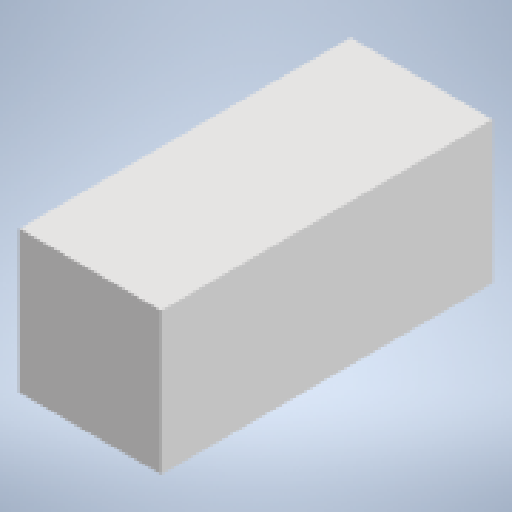
# Autodesk Inventor part: CalibrationPlate
Saved by Autodesk Inventor 2024 (Build 280153000, 153)
## iProperties
Created: 2023-12-31
Part Number: CalibrationPlate
Material: Generic
Document SubType Name: Modeling
Designer: jevan
Density: 1 g/cm^3
Appearance: Default
Author: jevan
Autodesk Inventor part; units mm, degrees
ref_plane "YZ Plane" through (0, 0, 0) normal (1, 0, 0) x (0, 1, 0)
ref_plane "XZ Plane" through (0, 0, 0) normal (0, 1, 0) x (-1, 0, 0)
ref_plane "XY Plane" through (0, 0, 0) normal (0, 0, 1) x (1, 0, 0)
sketch "Sketch1" plane through (0, 0, 0) normal (0, 1, 0) x (-1, 0, 0)
  line L0 (0, 0) -> (30, 0)
  line L1 (30, 0) -> (30, -70)
  line L2 (30, -70) -> (0, -70)
  line L3 (0, -70) -> (0, 0)
  dimension "d0" = 70
  dimension "d1" = 30
  constraints: 8 end point, 2 parallel, 1 horizontal, 1 perpendicular
  measures "d0" distance between parallel lines of L0 L2
  measures "d1" distance between parallel lines of L3 L1
extrude "Extrusion1" add sketch "Sketch1" along normal blind 30
sketch "Sketch2" plane through (0, 30, 0) normal (0, 1, 0) x (1, 0, 0)
  line L0 (-30, 70) -> (-30, 0) projected
  line L1 (0, 70) -> (-30, 70) projected
  line L2 (-30, 0) -> (0, 0)
  line L3 (0, 0) -> (0, 70)
  line L4 (0, 70) -> (-30, 70)
  line L5 (-30, 70) -> (-30, 0)
  line L6 (-6.75, 6.75) -> (-23.25, 6.75)
  line L7 (-23.25, 6.75) -> (-23.25, 63.25)
  line L8 (-23.25, 63.25) -> (-6.75, 63.25)
  line L9 (-6.75, 63.25) -> (-6.75, 6.75)
  dimension "d4" = 16.5
  constraints: 16 end point, 4 parallel, 2 perpendicular, 1 horizontal, 3 other
  measures "d4" distance between parallel lines of L9 L7
extrude "Extrusion2" cut sketch "Sketch2" against normal blind 10 contours L6 L7 L8 L9
chamfer "Chamfer1" distance 10 angle 60 1 edges at (-15, 20, -63.25) measured on face at (-12.25, 23.3333, -63.25)
chamfer "Chamfer3" distance 10 angle 60 1 edges at (-15, 20, -6.75) measured on face at (-17.75, 23.3333, -6.75)
move faces "Move1" translate (0, -7.938, 0) faces at (-12.25, 20, -38.6432)
move faces "Move2" translate (0, 13, 0) faces at (-20, 0, -46.6667)
chamfer "Chamfer4" distance 2 angle 45 4 edges at (-15, 13, 0) (0, 13, -35) (-30, 13, -35) (-15, 13, -70)
fillet "Fillet1" radius 5 12 edges at (-30, 22.5, 0) (0, 22.5, 0) (0, 22.5, -70) (-30, 22.5, -70) (-15, 30, 0) (-30, 30, -35) (-15, 30, -70) (0, 30, -35) (-15, 15, 0) (0, 15, -35) (-15, 15, -70) (-30, 15, -35)
body "Solid1"
